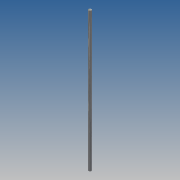
# Autodesk Inventor part: 10mm_Alu_Linearwelle_500mm
Saved by Autodesk Inventor 2015 SP1 (Build 190203100, 203)
## iProperties
Created: 2015-03-04
Part Number: 10mm_Alu_Linearwelle_500mm
Material: Aluminum 6061-AHC
Document SubType Name: Modeling
Designer: Marc
Mass: 106.025 g
Surface Area: 158.576 cm^2
Volume: 39.2687 cm^3
Density: 2.7 g/cm^3
Appearance: Aluminium - dunkel
Author: Marc
Autodesk Inventor part; units mm, degrees
ref_plane "YZ Plane" through (0, 0, 0) normal (1, 0, 0) x (0, 1, 0)
ref_plane "XZ Plane" through (0, 0, 0) normal (0, 1, 0) x (-1, 0, 0)
ref_plane "XY Plane" through (0, 0, 0) normal (0, 0, 1) x (1, 0, 0)
sketch "Skizze1" plane through (0, 0, 0) normal (0, 0, 1) x (1, 0, 0)
  line L0 (0, -7) -> (0, 7) projected
  line L1 (-7, 0) -> (7, 0) projected
  circle A0 centre (0, 0) radius 5
  dimension "d0" = 10
  constraints: 1 centre point, 1 coincident
  measures "d0" diameter of A0
extrude "Extrusion1" add sketch "Skizze1" along normal mid plane 500
chamfer "Fase1" distance 0.2 angle 45 1 edges at (-5, 0, 250)
chamfer "Fase2" distance 0.2 angle 45 1 edges at (-5, 0, -250)
